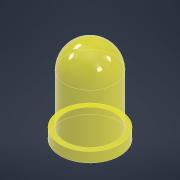
# Autodesk Inventor part: LED5mm
Saved by Autodesk Inventor 2022.2 (Build 262287000, 287)
## iProperties
Created: 2023-05-21
Part Number: LED5mm
Material: Glass
Document SubType Name: Modeling
Designer: jaege
Density: 2.18 g/cm^3
Appearance: Clear - Yellow - Opaque
Author: jaege
Autodesk Inventor part; units mm, degrees
ref_plane "YZ Plane" through (0, 0, 0) normal (1, 0, 0) x (0, 1, 0)
ref_plane "XZ Plane" through (0, 0, 0) normal (0, 1, 0) x (-1, 0, 0)
ref_plane "XY Plane" through (0, 0, 0) normal (0, 0, 1) x (1, 0, 0)
sketch "Sketch1" plane through (0, 0, 0) normal (0, 1, 0) x (-1, 0, 0)
  circle A0 centre (0, 0) radius 3
  dimension "d0" = 6
  constraints: 1 centre point, 1 coincident
  measures "d0" diameter of A0
extrude "Extrusion1" add sketch "Sketch1" along normal blind 1
sketch "Sketch2" plane through (0, 1, 0) normal (0, 1, 0) x (1, 0, 0)
  circle A0 centre (0, 0) radius 2.5
  dimension "d3" = 5
  constraints: 1 centre point, 1 coincident
  measures "d3" diameter of A0
extrude "Extrusion2" add sketch "Sketch2" along normal blind 5
sketch "Sketch4" plane through (0, 0, 0) normal (1, 0, 0) x (0, 1, 0)
  line L0 (6, -2.5) -> (6, 2.5) projected
  line L1 (1, 2.5) -> (1, -2.5) projected
  line L2 (1, 2.5) -> (6, 2.5) projected
  line L3 (6, -2.5) -> (6, 2.5) projected
  arc A0 (8.5, 0) -> (6, 2.5) centre (6, 0) ccw
  line L4 (8.5, 0) -> (6, 0)
  point P0 (0, 0)
  constraints: 2 end point, 2 point on circle, 1 centre point, 1 midpoint, 1 perpendicular
revolve "Revolution1" add sketch "Sketch4" angle 360 about axis through (0, 8.5, 0) along (0, -1, 0)
body "Solid1"
